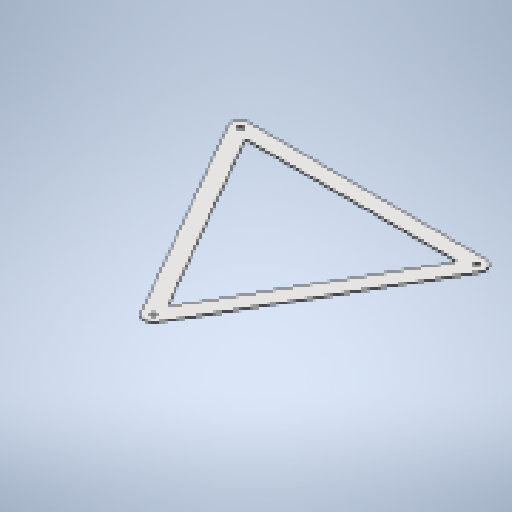
# Autodesk Inventor part: PNS-689 leg floor pattern
Saved by Autodesk Inventor 2025.1 (Build 291241020, 241B)
## iProperties
Created: 2025-02-20
Part Number: PNS-689 leg floor pattern
Material: Stainless Steel
Document SubType Name: Sheet Metal
Designer: user
Mass: 1070.67 g
Surface Area: 320.872 cm^2
Volume: 133.833 cm^3
Density: 8 g/cm^3
Flat Pattern Width: 69.8266 cm
Flat Pattern Length: 79.747 cm
Flat Pattern Area: 5568.46 cm^2
Sheet Metal Rule: AISI304 3mm Die 32
Sheet Metal Width: 698.266 mm
Sheet Metal Length: 797.470 mm
Sheet Metal Area: 556846.052 mm^2
Appearance: Default
Author: user
Autodesk Inventor part; units mm, degrees
ref_plane "YZ Plane" through (0, 0, 0) normal (1, 0, 0) x (0, 1, 0)
ref_plane "XZ Plane" through (0, 0, 0) normal (0, 1, 0) x (-1, 0, 0)
ref_plane "XY Plane" through (0, 0, 0) normal (0, 0, 1) x (1, 0, 0)
sketch "Sketch1" plane through (0, 0, 0) normal (0, 0, 1) x (1, 0, 0)
  circle A0 centre (0, 0) radius 8.5
  line L0 (-394.9167, 627.0158) -> (-24.6817, -14.25)
  arc A1 (-24.6817, -14.25) -> (24.6817, -14.25) centre (0, 0) ccw
  line L1 (24.6817, -14.25) -> (394.9167, 627.0158)
  arc A2 (394.9167, 627.0158) -> (370.235, 669.7658) centre (370.235, 641.2658) ccw
  line L2 (370.235, 669.7658) -> (-370.235, 669.7658)
  arc A3 (-370.235, 669.7658) -> (-394.9167, 627.0158) centre (-370.235, 641.2658) ccw
  line L3 (0, 0) -> (0, 669.7658) construction
  line L4 (-332.9959, 619.7658) -> (332.9959, 619.7658)
  line L5 (332.9959, 619.7658) -> (0, 43)
  line L6 (0, 43) -> (-332.9959, 619.7658)
  circle A4 centre (-370.235, 641.2658) radius 8.5
  circle A5 centre (370.235, 641.2658) radius 8.5
  dimension "d34" = 17
  dimension "d35" = 20
  dimension "d36" = 740.47
  dimension "d37" = 740.47
  dimension "d38" = 50
  measures "d34" diameter of A0
  measures "d35" radial gap between concentric circles of A1 A0
  measures "d36" distance of A3.centre A2.centre
  measures "d37" distance of L3.start A2.centre
  measures "d38" distance between parallel lines of L2 L4
extrude "Plate1" add sketch "Sketch1" along normal blind 3
fillet "Corner Round3" radius 6 3 edges at (-332.9959, 619.7658, 1.5) (0, 43, 1.5) (332.9959, 619.7658, 1.5)
equation "\"d37\" = d36"
equation "\"d2\" = Thickness"
equation "\"BendReliefWidth\" = Thickness"
equation "\"BendReliefDepth\" = 0.5 * Thickness"
equation "\"CornerReliefSize\" = 4 * Thickness"
equation "\"MinimumRemnant\" = 2 * Thickness"
equation "\"TransitionRadius\" = BendRadius"
equation "\"JacobiRadiusSize\" = BendRadius"
equation "\"GapSize\" = Thickness"
equation "\"Thickness\" = 3"
equation "\"BendRadius\" = 5"
body "Solid1"
